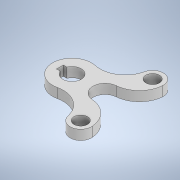
# Autodesk Inventor part: Part5
Saved by Autodesk Inventor 2021 (Build 250183000, 183)
## iProperties
Created: 2022-04-24
Part Number: Part5
Material: Generic
Document SubType Name: Modeling
Designer: hp
Density: 1 g/cm^3
Appearance: Default
Author: hp
Autodesk Inventor part; units mm, degrees
ref_plane "YZ Plane" through (0, 0, 0) normal (1, 0, 0) x (0, 1, 0)
ref_plane "XZ Plane" through (0, 0, 0) normal (0, 1, 0) x (-1, 0, 0)
ref_plane "XY Plane" through (0, 0, 0) normal (0, 0, 1) x (1, 0, 0)
sketch "Sketch1" plane through (0, 0, 0) normal (0, 1, 0) x (-1, 0, 0)
  arc A0 (148.5653, -569.1641) -> (148.5653, -373.8126) centre (170, -471.4884) ccw
  arc A1 (4.7545, -533.3058) -> (4.7545, -409.6709) centre (0, -471.4884) ccw
  arc A2 (-6.2783, -274.6993) -> (-114.7972, -291.2071) centre (-60, -286.4884) ccw
  arc A3 (-114.7972, -651.7696) -> (-6.2783, -668.2775) centre (-60, -656.4884) ccw
  arc A4 (-6.2783, -274.6993) -> (148.5653, -373.8126) centre (120.7001, -246.8341) ccw
  arc A5 (148.5653, -569.1641) -> (-6.2783, -668.2775) centre (120.7001, -696.1426) ccw
  arc A6 (-114.7972, -291.2071) -> (4.7545, -409.6709) centre (14.7235, -280.0537) ccw
  arc A7 (4.7545, -533.3058) -> (-114.7972, -651.7696) centre (14.7235, -662.923) ccw
  circle A8 centre (-60, -286.4884) radius 35
  arc A9 (214.1588, -453.9884) -> (214.1588, -488.9884) centre (170, -471.4884) ccw
  circle A10 centre (-60, -656.4884) radius 35
  line L0 (232.5, -453.9884) -> (214.1588, -453.9884)
  line L1 (214.1588, -488.9884) -> (232.5, -488.9884)
  line L2 (232.5, -488.9884) -> (232.5, -453.9884)
  point P0 (0, 0)
  dimension "d0" = 200
  dimension "d1" = 124
  dimension "d2" = 170
  dimension "d3" = 110
  dimension "d4" = 110
  dimension "d5" = 370
  dimension "d6" = 185
  dimension "d7" = 260
  dimension "d8" = 230
  dimension "d9" = 0
  dimension "d10" = 260
  dimension "d11" = 0
  dimension "d12" = 260
  dimension "d13" = 260
  dimension "d14" = 70
  dimension "d15" = 70
  dimension "d16" = 95
  dimension "d17" = 35
  dimension "d18" = 17.5
  dimension "d19" = 62.5
  constraints: 18 point on circle, 11 centre point, 8 tangent, 6 end point, 3 coincident, 1 horizontal, 1 parallel
  measures "d0" diameter of A0
  measures "d1" diameter of A1
  measures "d2" distance of A1.centre A0.centre
  measures "d3" diameter of A2
  measures "d4" diameter of A3
  measures "d5" distance of A3.centre A2.centre
  measures "d6" vertical distance of A3.centre A1.centre
  measures "d7" diameter of A4
  measures "d8" horizontal distance of A0.centre A3.centre
  measures "d9" vertical distance of A0.centre A1.centre
  measures "d10" diameter of A5
  measures "d11" horizontal distance of A3.centre A2.centre
  measures "d12" diameter of A6
  measures "d13" diameter of A7
  measures "d14" diameter of A8
  measures "d15" diameter of A10
  measures "d16" diameter of A9
  measures "d17" distance of L1.end L0.start
  measures "d18" distance from line of A0.centre L1
  measures "d19" distance from line of L2 A0.centre
extrude "Extrusion1" add sketch "Sketch1" along normal blind 50
equation "\"d4\" = d3"
equation "\"d6\" = 0.5 * d5"
equation "\"d10\" = d7"
equation "\"d18\" = 0.5 * d17"
body "Solid1"
